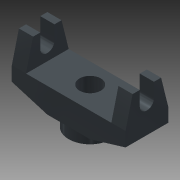
# Autodesk Inventor part: HW 7 Part 1
Saved by Autodesk Inventor 2015 (Build 190159000, 159)
## iProperties
Created: 2016-02-24
Part Number: HW 7 Part 1
Material: Iron, Cast
Document SubType Name: Modeling
Designer: Melissa
Density: 7.15 g/cm^3
Appearance: Iron Gray
Mass: 5210.81 g
Surface Area: 774.468 cm^2
Volume: 728.785 cm^3
Author: Melissa
Autodesk Inventor part; units mm, degrees
ref_plane "YZ Plane" through (0, 0, 0) normal (1, 0, 0) x (0, 1, 0)
ref_plane "XZ Plane" through (0, 0, 0) normal (0, 1, 0) x (-1, 0, 0)
ref_plane "XY Plane" through (0, 0, 0) normal (0, 0, 1) x (1, 0, 0)
sketch "Sketch1" plane through (0, 0, 0) normal (0, 0, 1) x (1, 0, 0)
  line L0 (0, 0) -> (0, 25.4)
  line L1 (0, 25.4) -> (-203.2, 25.4)
  line L2 (-203.2, 25.4) -> (-203.2, 0)
  line L3 (-203.2, 0) -> (-139.7, -19.05)
  line L4 (-139.7, -19.05) -> (-63.5, -19.05)
  line L5 (-63.5, -19.05) -> (0, 0)
  dimension "d0" = 203.2
  dimension "d1" = 25.4
  dimension "d2" = 63.5
  dimension "d3" = 44.45
  constraints: 12 end point, 2 equal length, 2 perpendicular, 1 parallel, 1 vertical
  measures "d0" distance of L0.end L1.end
  measures "d1" distance of L0.start L0.end
  measures "d2" horizontal distance of L3.end L2.end
  measures "d3" distance between parallel lines of L4 L1
extrude "Extrusion1" add sketch "Sketch1" against normal blind 76.2
sketch "Sketch2" plane through (0, 0, 0) normal (1, 0, 0) x (0, 0, -1)
  line L0 (12.7, 76.2) -> (25.4, 76.2)
  line L1 (25.4, 76.2) -> (25.4, 50.8)
  line L2 (76.2, 25.4) -> (63.5, 76.2)
  line L3 (63.5, 76.2) -> (50.8, 76.2)
  line L4 (0, 25.4) -> (76.2, 25.4) projected
  line L5 (50.8, 76.2) -> (50.8, 50.8)
  arc A0 (25.4, 50.8) -> (50.8, 50.8) centre (38.1, 50.8) ccw
  line L6 (0, 25.4) -> (12.7, 76.2)
  line L7 (0, 25.4) -> (76.2, 25.4)
  point P0 (0, 0)
  dimension "d6" = 12.7
  dimension "d7" = 25.4
  dimension "d8" = 76.2
  dimension "d9" = 76.2
  dimension "d10" = 50.8
  constraints: 14 end point, 2 equal length, 2 horizontal, 2 perpendicular, 2 point on circle, 2 tangent, 1 centre point, 1 parallel
  measures "d6" radius of A0
  measures "d7" horizontal distance of A0.centre L2.end
  measures "d8" vertical distance of point (0, 0) L0.start
  measures "d9" vertical distance of point (0, 0) L2.end
  measures "d10" distance of L2.end L0.start
extrude "Extrusion2" add sketch "Sketch2" against normal blind 203.2
sketch "Sketch3" plane through (0, 76.2, -12.7) normal (0, 1, 0) x (1, 0, 0)
  line L0 (0, -12.7) -> (-203.2, -12.7) projected
  line L1 (-177.8, -12.7) -> (-177.8, 63.5)
  line L2 (-139.7, 63.5) -> (-203.2, 63.5) projected
  line L3 (-177.8, -12.7) -> (-25.4, -12.7)
  line L4 (-63.5, -12.7) -> (0, -12.7) projected
  line L5 (-25.4, -12.7) -> (-25.4, 63.5)
  line L6 (0, 63.5) -> (-63.5, 63.5) projected
  line L7 (-25.4, 63.5) -> (-177.8, 63.5)
  line L8 (-203.2, 12.7) -> (-203.2, 38.1) projected
  line L9 (0, 38.1) -> (0, 12.7) projected
  dimension "d13" = 25.4
  dimension "d14" = 25.4
  constraints: 8 end point, 4 point on line, 2 vertical, 1 collinear
  measures "d13" distance between parallel lines of L8 L1
  measures "d14" distance between parallel lines of L9 L5
extrude "Extrusion3" cut sketch "Sketch3" against normal blind 50.8
sketch "Sketch4" plane through (-139.7, -19.05, 0) normal (0, -1, 0) x (1, 0, 0)
  circle A0 centre (38.1, -38.1) radius 38.1
  line L0 (0, 0) -> (76.2, 0) projected
  line L1 (76.2, 0) -> (76.2, -76.2) projected
  point P0 (139.7, 0)
  dimension "d17" = 76.2
  constraints: 2 tangent, 1 centre point
  measures "d17" diameter of A0
extrude "Extrusion4" add sketch "Sketch4" along normal blind 19.05 contours A0
hole "Hole1" at (-103.5367, -38.1, -40.3531) direction (0, 1, 0) diameter 38.1 end through all
body "Solid1"
